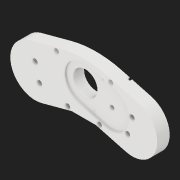
# Autodesk Inventor part: HA002
Saved by Autodesk Inventor 2017 SP1 (Build 210196100, 196)
## iProperties
Created: 2017-06-10
Part Number: HA002
Material: ABS Plastic
Document SubType Name: Modeling
Designer: Zach
Density: 1.06 g/cm^3
Appearance: CR White
Author: Zach
Autodesk Inventor part; units mm, degrees
ref_plane "XZ Plane" through (0, 0, 0) normal (0, 1, 0) x (-1, 0, 0)
ref_plane "XY Plane" through (0, 0, 0) normal (0, 0, 1) x (1, 0, 0)
sketch "Sketch1" plane through (0, 0, 0) normal (0, 0, 1) x (1, 0, 0)
  line L0 (0, 0) -> (160, 0)
  line L1 (160, 0) -> (118.589, -154.5481)
  line L2 (0, 0) -> (41.411, -154.5481)
  line L3 (41.411, -154.5481) -> (118.589, -154.5481)
  dimension "d0" = 160
  dimension "d1" = 160
  dimension "d2" = 160
  dimension "d3" = 75
  dimension "d4" = 75
  constraints: 8 end point, 1 coincident, 1 horizontal
  measures "d0" distance of L0.start L0.end
  measures "d1" distance of L0.end L1.end
  measures "d2" distance of L0.start L2.end
  measures "d3" angle of L0 L1
  measures "d4" angle of L0 L2
extrude "Extrusion1" add sketch "Sketch1" along normal blind 40
sketch "Sketch5" plane through (0, 0, 40) normal (0, 0, 1) x (1, 0, 0)
  line L0 (160, 0) -> (0, 0) projected
  line L1 (160, 0) -> (256.5926, -25.8819)
  line L2 (118.589, -154.5481) -> (41.411, -154.5481) projected
  line L3 (118.589, -154.5481) -> (215.1815, -180.43)
  circle A0 centre (235.8871, -103.156) radius 80 construction
  arc A1 (215.1815, -180.43) -> (256.5926, -25.8819) centre (235.8871, -103.156) ccw
  line L4 (160, 0) -> (118.589, -154.5481)
  line L5 (0, 0) -> (41.411, -154.5481) projected
  line L6 (0, 0) -> (-96.5926, -25.8819)
  line L7 (41.411, -154.5481) -> (118.589, -154.5481) projected
  line L8 (41.411, -154.5481) -> (-55.1815, -180.43)
  circle A2 centre (-75.8871, -103.156) radius 80 construction
  arc A3 (-96.5926, -25.8819) -> (-55.1815, -180.43) centre (-75.8871, -103.156) ccw
  point P0 (90, 0)
  dimension "d25" = 100
  dimension "d26" = 100
  dimension "d27" = 160
  dimension "d30" = 100
  dimension "d31" = 100
  dimension "d32" = 160
  constraints: 10 end point, 8 point on circle, 6 tangent, 4 centre point, 1 concentric
  measures "d25" distance of L0.start L1.end
  measures "d26" distance of L2.start L3.end
  measures "d27" diameter of A0
  measures "d30" distance of L0.end L6.end
  measures "d31" distance of L2.end L8.end
  measures "d32" diameter of A2
extrude "Extrusion5" add sketch "Sketch5" against normal blind 40 contours L1 A1 L3 L4 | L5 L8 A3 L6
sketch "Sketch7" plane through (0, 0, 40) normal (0, 0, 1) x (1, 0, 0)
  line L0 (-75.7601, -74.6519) -> (-61.5251, -127.7778) construction
  line L1 (-68.6426, -101.2148) -> (20.7055, -77.2741) construction
  circle A0 centre (-75.7601, -74.6519) radius 2.5
  circle A1 centre (-61.5251, -127.7778) radius 2.5
  line L2 (0, 0) -> (-96.5926, -25.8819) construction
  line L3 (-55.1815, -180.43) -> (41.411, -154.5481) construction
  line L4 (-96.5926, -25.8819) -> (0, 0) construction
  line L5 (0, 0) -> (41.411, -154.5481) construction
  line L6 (41.411, -154.5481) -> (-55.1815, -180.43) construction
  line L7 (160, 0) -> (256.5926, -25.8819) construction
  line L8 (215.1815, -180.43) -> (118.589, -154.5481) construction
  line L9 (118.589, -154.5481) -> (160, 0) construction
  line L10 (139.2945, -77.2741) -> (228.6426, -101.2148) construction
  line L11 (221.5251, -127.7778) -> (235.7601, -74.6519) construction
  circle A2 centre (235.7601, -74.6519) radius 2.5
  circle A3 centre (221.5251, -127.7778) radius 2.5
  dimension "d35" = 55
  dimension "d37" = 5
  dimension "d38" = 5
  dimension "d46" = 92.5
  dimension "d47" = 92.5
  dimension "d48" = 55
  dimension "d49" = 5
  dimension "d50" = 5
  constraints: 12 end point, 6 perpendicular, 4 centre point, 4 coincident, 4 midpoint, 1 point on line
  measures "d35" distance of L0.start L0.end
  measures "d37" diameter of A0
  measures "d38" diameter of A1
  measures "d46" distance of L1.end L1.start
  measures "d47" distance of L10.end L10.start
  measures "d48" distance of L11.start L11.end
  measures "d49" diameter of A2
  measures "d50" diameter of A3
extrude "Extrusion7" cut sketch "Sketch7" against normal through all
sketch "Sketch8" plane through (0, 0, 40) normal (0, 0, 1) x (1, 0, 0)
  circle A0 centre (-75.7601, -74.6519) radius 2.5 projected
  circle A1 centre (-61.5251, -127.7778) radius 2.5 projected
  circle A2 centre (-75.7601, -74.6519) radius 7.5
  circle A3 centre (-61.5251, -127.7778) radius 7.5
  circle A4 centre (235.7601, -74.6519) radius 2.5 projected
  circle A5 centre (221.5251, -127.7778) radius 2.5 projected
  circle A6 centre (235.7601, -74.6519) radius 7.5
  circle A7 centre (221.5251, -127.7778) radius 7.5
  point P0 (0, 0)
  dimension "d42" = 15
  dimension "d43" = 15
  dimension "d51" = 15
  dimension "d52" = 15
  constraints: 4 centre point, 4 coincident
  measures "d42" diameter of A2
  measures "d43" diameter of A3
  measures "d51" diameter of A6
  measures "d52" diameter of A7
extrude "Extrusion8" cut sketch "Sketch8" against normal blind 30 contours A2 | A3 | A4 | A5 | A6 | A7
sketch "Sketch9" plane through (0, 0, 40) normal (0, 0, 1) x (1, 0, 0)
  circle A0 centre (80, -60) radius 39
  line L0 (41.411, -154.5481) -> (118.589, -154.5481) projected
  point P0 (0, 0)
  point P1 (80, -154.5481)
  dimension "d53" = 78
  dimension "d54" = 60
  constraints: 1 centre point, 1 midpoint, 1 vertical alignment
  measures "d53" diameter of A0
  measures "d54" vertical distance of A0.centre point (0, 0)
extrude "Extrusion9" cut sketch "Sketch9" against normal through all
sketch "Sketch10" plane through (0, 0, 40) normal (0, 0, 1) x (1, 0, 0)
  circle A0 centre (80, -304.672) radius 315 construction
  line L0 (160, 0) -> (0, 0) projected
  arc A1 (160, 0) -> (0, 0) centre (80, -304.672) ccw
  dimension "d57" = 630
  constraints: 4 point on circle, 2 centre point, 1 concentric
  measures "d57" diameter of A0
extrude "Extrusion10" add sketch "Sketch10" against normal blind 40
sketch "Sketch11" plane through (0, 0, 40) normal (0, 0, 1) x (1, 0, 0)
  circle A0 centre (-6.7279, -84.0474) radius 60 construction
  circle A1 centre (80, -60) radius 60 construction
  line L0 (-22.7595, -26.2289) -> (63.9684, -2.1814)
  line L1 (9.3038, -141.866) -> (96.0316, -117.8186)
  arc A2 (96.0316, -117.8186) -> (63.9684, -2.1814) centre (80, -60) ccw
  arc A3 (-22.7595, -26.2289) -> (9.3038, -141.866) centre (-6.7279, -84.0474) ccw
  circle A4 centre (-75.7601, -74.6519) radius 2.5 construction
  circle A5 centre (-61.5251, -127.7778) radius 2.5 construction
  line L2 (-75.7601, -74.6519) -> (-61.5251, -127.7778) construction
  line L3 (-68.6426, -101.2148) -> (80, -60) construction
  point P0 (0, 0)
  dimension "d60" = 120
  dimension "d61" = 90
  dimension "d68" = 120
  constraints: 8 end point, 8 point on circle, 6 tangent, 4 centre point, 2 coincident, 1 concentric, 1 midpoint, 1 point on line
  measures "d60" diameter of A0
  measures "d61" distance of point (80, -60) A0.centre
  measures "d68" diameter of A1
extrude "Extrusion11" cut sketch "Sketch11" against normal blind 5
sketch "Sketch12" plane through (0, 0, 35) normal (0, 0, 1) x (1, 0, 0)
  circle A0 centre (-6.7279, -84.0474) radius 6.5
  arc A1 (-22.7595, -26.2289) -> (9.3038, -141.866) centre (-6.7279, -84.0474) ccw projected
  point P0 (0, 0)
  dimension "d64" = 13
  constraints: 1 centre point, 1 coincident
  measures "d64" diameter of A0
extrude "Extrusion12" cut sketch "Sketch12" against normal through all
sketch "Sketch13" plane through (0, 0, 0) normal (0, 0, -1) x (-1, 0, 0)
  circle A0 centre (6.7279, -84.0474) radius 6.5 construction
  line L0 (1.6217, -67.844) -> (-5.9934, -95.3078)
  line L1 (-5.9934, -95.3078) -> (11.834, -100.2509)
  line L2 (11.834, -100.2509) -> (19.4491, -72.7871)
  line L3 (19.4491, -72.7871) -> (1.6217, -67.844)
  line L4 (1.6217, -67.844) -> (11.834, -100.2509) construction
  line L5 (-5.9934, -95.3078) -> (19.4491, -72.7871) construction
  line L6 (-1.7631, -69.7592) -> (21.3643, -76.1719)
  line L7 (21.3643, -76.1719) -> (15.2188, -98.3357)
  line L8 (15.2188, -98.3357) -> (-7.9086, -91.923)
  line L9 (-7.9086, -91.923) -> (-1.7631, -69.7592)
  line L10 (-1.7631, -69.7592) -> (15.2188, -98.3357) construction
  line L11 (21.3643, -76.1719) -> (-7.9086, -91.923) construction
  line L12 (18.6924, -85.8083) -> (17.8908, -88.6992)
  line L13 (17.8908, -88.6992) -> (19.8181, -89.2336)
  line L14 (19.8181, -89.2336) -> (20.6196, -86.3427)
  line L15 (20.6196, -86.3427) -> (18.6924, -85.8083)
  line L16 (-4.4066, -83.0356) -> (-3.3378, -79.181)
  line L17 (-3.3378, -79.181) -> (-0.4469, -79.9826)
  line L18 (-0.4469, -79.9826) -> (-1.5157, -83.8372)
  line L19 (-1.5157, -83.8372) -> (-4.4066, -83.0356)
  line L20 (-3.8722, -81.1083) -> (-4.8359, -80.8411) construction
  line L21 (-0.9813, -81.9099) -> (6.7279, -84.0474) construction
  circle A1 centre (6.7279, -84.0474) radius 6.5 projected
  circle A2 centre (-80, -60) radius 39 construction
  line L22 (-80, -60) -> (6.7279, -84.0474) construction
  point P0 (0, 0)
  point P1 (18.2916, -87.2538)
  point P2 (-4.354, -80.9747)
  dimension "d69" = 28.5
  dimension "d70" = 18.5
  dimension "d71" = 23
  dimension "d72" = 24
  dimension "d73" = 2
  dimension "d74" = 3
  dimension "d75" = 3
  dimension "d76" = 4
  dimension "d77" = 8
  constraints: 46 end point, 11 midpoint, 9 parallel, 6 perpendicular, 3 point on line, 1 centre point, 1 coincident
  measures "d69" distance of L3.end L1.start
  measures "d70" distance of L1.start L1.end
  measures "d71" distance of L11.start L8.start
  measures "d72" distance of L8.start L8.end
  measures "d73" distance of L13.end L13.start
  measures "d74" distance of L13.end L15.start
  measures "d75" distance of L18.start L16.end
  measures "d76" distance of L18.start L18.end
  measures "d77" distance of L21.start L21.end
extrude "Extrusion13" cut sketch "Sketch13" against normal blind 21 contours L3 L2 L6 L0 | L6 L2 L8 L0 L19 L18 L17 | L0 L17 L16 L19 L8 L9 L6 | L17 L18 L19 L0 | L6 L7 L8 L2 | L2 L1 L0 L8 | L15 L14 L13 L7 | A1
sketch "Sketch14" plane through (0, 0, 0) normal (0, 0, -1) x (-1, 0, 0)
  line L0 (-1.6515, -79.6486) -> (-3.3378, -79.181) projected
  line L1 (-3.3378, -79.181) -> (-4.4066, -83.0356) projected
  line L2 (-4.4066, -83.0356) -> (-2.7202, -83.5032) projected
  line L3 (-2.7202, -83.5032) -> (-1.6515, -79.6486) projected
  point P0 (0, 0)
extrude "Extrusion14" cut sketch "Sketch14" against normal blind 24
sketch "Sketch15" plane through (-11.834, -100.2509, 21) normal (-0.2671937, 0.9636428, 0) x (0.9636428, 0.2671937, 0)
  circle A0 centre (5.6915, 16.5) radius 4
  line L0 (9.6915, 16.5) -> (9.6915, 21)
  line L1 (1.6915, 21) -> (1.6915, 16.5)
  line L2 (0, 21) -> (18.5, 21) projected
  line L3 (0, 21) -> (0, 0) construction
  line L4 (0, 0) -> (18.5, 0) construction
  line L5 (18.5, 21) -> (18.5, 0) construction
  line L6 (9.25, 0) -> (9.25, 21) construction
  line L7 (9.6915, 21) -> (1.6915, 21)
  line L8 (36.8014, 21) -> (-63.1949, 21) projected
  point P0 (38.1902, 21)
  point P1 (9.25, 21)
  dimension "d82" = 8
  dimension "d87" = 3.5585
  dimension "d88" = 4.5
  constraints: 8 end point, 2 midpoint, 2 point on circle, 2 point on line, 2 tangent, 2 vertical, 1 centre point, 1 collinear, 1 perpendicular
  measures "d82" diameter of A0
  measures "d87" distance from line of A0.centre L6
  measures "d88" distance from line of L2 A0.centre
extrude "Extrusion15" cut sketch "Sketch15" along normal through all
sketch "Sketch16" plane through (0, 0, 35) normal (0, 0, 1) x (1, 0, 0)
  line L0 (96.0316, -117.8186) -> (9.3038, -141.866) construction
  line L1 (-22.7595, -26.2289) -> (63.9684, -2.1814) construction
  line L2 (52.6677, -129.8423) -> (20.6044, -14.2051) construction
  line L3 (50.6637, -122.615) -> (22.6084, -21.4325) construction
  circle A0 centre (50.6637, -122.615) radius 1.5
  circle A1 centre (22.6084, -21.4325) radius 1.5
  point P0 (0, 0)
  point P1 (36.6361, -72.0237)
  dimension "d89" = 105
  dimension "d90" = 3
  dimension "d91" = 3
  constraints: 4 end point, 4 midpoint, 2 centre point, 2 coincident, 2 point on line
  measures "d89" distance of L3.end L3.start
  measures "d90" diameter of A0
  measures "d91" diameter of A1
extrude "Extrusion16" cut sketch "Sketch16" against normal blind 25
sketch "Sketch17" plane through (0, 0, 40) normal (0, 0, 1) x (1, 0, 0)
  circle A0 centre (80, -60) radius 39 projected
  point P0 (0, 0)
ref_plane "Work Plane1" through (80, -60, 40) normal (1, 0, 0) x (0, 1, 0)
mirror "Mirror1" about plane through (80, -60, 40) normal (1, 0, 0) of "Extrusion1", "Extrusion5", "Extrusion7", "Extrusion8", "Extrusion9", "Extrusion10", "Extrusion11", "Extrusion12", "Extrusion13", "Extrusion14", "Extrusion15", "Extrusion16"
sketch "Sketch18" plane through (0, 0, 40) normal (0, 0, 1) x (1, 0, 0)
  line L0 (160, 0) -> (187.5287, -7.3763) construction
  line L1 (160, 0) -> (118.589, -154.5481) construction
  line L2 (41.411, -154.5481) -> (118.589, -154.5481) construction
  line L3 (0, 0) -> (41.411, -154.5481) construction
  circle A0 centre (29.0657, -147.1117) radius 2.5
  circle A1 centre (130.9343, -147.1117) radius 2.5
  line L4 (130.9343, -147.1117) -> (121.275, -144.5235) construction
  line L5 (29.0657, -147.1117) -> (38.725, -144.5235) construction
  line L6 (63.9684, -117.8186) -> (150.6962, -141.866) construction
  line L7 (138.514, -138.4882) -> (132.991, -158.4071) construction
  line L8 (130.9343, -147.1117) -> (135.7525, -148.4477) construction
  line L9 (215.1815, -180.43) -> (118.589, -154.5481) construction
  circle A2 centre (-7.1585, -11.9211) radius 2.5
  circle A3 centre (167.1585, -11.9211) radius 2.5
  line L10 (182.7595, -26.2289) -> (96.0316, -2.1814) projected
  line L11 (167.1585, -11.9211) -> (157.4993, -9.3329) construction
  line L12 (167.1585, -11.9211) -> (171.9881, -13.2152) construction
  line L13 (169.4064, -22.5264) -> (174.5699, -3.904) construction
  line L14 (-7.1585, -11.9211) -> (2.5007, -9.3329)
  dimension "d94" = 5
  dimension "d95" = 5
  dimension "d96" = 10
  dimension "d97" = 5
  dimension "d98" = 5
  dimension "d99" = 5
  dimension "d102" = 10
  dimension "d103" = 5
  constraints: 20 end point, 9 point on line, 8 perpendicular, 4 centre point, 4 horizontal alignment, 2 midpoint
  measures "d94" diameter of A0
  measures "d95" diameter of A1
  measures "d96" distance of L4.start L4.end
  measures "d97" distance of L4.start L8.end
  measures "d98" diameter of A2
  measures "d99" diameter of A3
  measures "d102" distance of L11.start L11.end
  measures "d103" distance of L12.end L11.start
extrude "Extrusion17" cut sketch "Sketch18" against normal through all
sketch "Sketch19" plane through (-75.7601, -74.6519, 10) normal (0, 0, 1) x (1, 0, 0)
  circle A0 centre (68.6016, 62.7308) radius 2.5 projected
  circle A1 centre (104.8258, -72.4598) radius 2.5 projected
  circle A2 centre (206.6944, -72.4598) radius 2.5 projected
  circle A3 centre (242.9187, 62.7308) radius 2.5 projected
  circle A4 centre (68.6016, 62.7308) radius 2.5 projected
  circle A5 centre (68.6016, 62.7308) radius 7.5
  circle A6 centre (242.9187, 62.7308) radius 2.5 projected
  circle A7 centre (242.9187, 62.7308) radius 7.5
  circle A8 centre (206.6944, -72.4598) radius 2.5 projected
  circle A9 centre (206.6944, -72.4598) radius 7.5
  circle A10 centre (104.8258, -72.4598) radius 2.5 projected
  circle A11 centre (104.8258, -72.4598) radius 7.5
  point P0 (75.7601, 74.6519)
  dimension "d106" = 15
  dimension "d107" = 15
  dimension "d108" = 15
  dimension "d109" = 15
  constraints: 4 centre point, 4 coincident
  measures "d106" diameter of A5
  measures "d107" diameter of A7
  measures "d108" diameter of A9
  measures "d109" diameter of A11
extrude "Extrusion18" cut sketch "Sketch19" along normal through all
body "Solid1"
